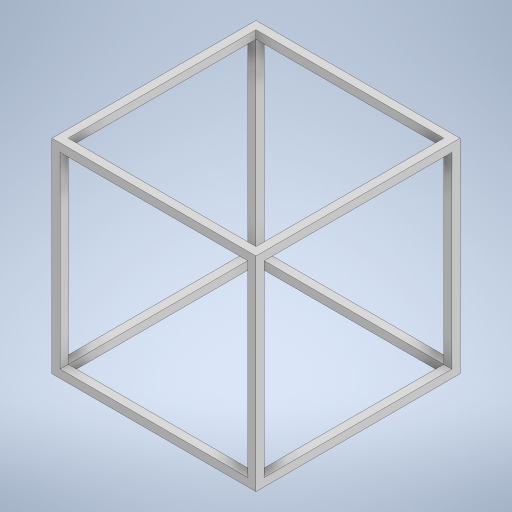
# Autodesk Inventor part: wymiar
Saved by Autodesk Inventor 2023.5 (Build 275446000, 446)
## iProperties
Created: 2025-03-17
Part Number: wymiar
Material: Ogólny
Document SubType Name: Modeling
Designer: kamil
Density: 1 g/cm^3
Appearance: Domyślna
Author: kamil
Autodesk Inventor part; units mm, degrees
ref_plane "YZ Plane" through (0, 0, 0) normal (1, 0, 0) x (0, 1, 0)
ref_plane "XZ Plane" through (0, 0, 0) normal (0, 1, 0) x (-1, 0, 0)
ref_plane "XY Plane" through (0, 0, 0) normal (0, 0, 1) x (1, 0, 0)
sketch "Szkic1" plane through (0, 0, 0) normal (0, 1, 0) x (-1, 0, 0)
  line L0 (0, 0) -> (-50, 0)
  line L1 (-50, 0) -> (-50, -50)
  line L2 (-50, -50) -> (0, -50)
  line L3 (0, -50) -> (0, 0)
  line L4 (-2, -2) -> (-48, -2)
  line L5 (-48, -2) -> (-48, -48)
  line L6 (-48, -48) -> (-2, -48)
  line L7 (-2, -48) -> (-2, -2)
  dimension "d0" = 50
  dimension "d1" = 50
  dimension "d2" = 2
  constraints: 16 end point, 4 parallel, 2 perpendicular, 1 horizontal, 3 other
  measures "d0" distance of L2.end L1.end
  measures "d1" distance of L2.end L0.start
  measures "d2" distance between parallel lines of L3 L7
extrude "Wyciągnięcie proste1" add sketch "Szkic1" along normal blind 2
sketch "Szkic2" plane through (0, 2, 0) normal (0, 1, 0) x (1, 0, 0)
  line L0 (50, 0) -> (50, 50) projected
  line L1 (50, 50) -> (0, 50) projected
  line L2 (0, 50) -> (0, 0) projected
  line L3 (0, 0) -> (50, 0) projected
  line L4 (2, 2) -> (2, 48) projected
  line L5 (2, 48) -> (48, 48) projected
  line L6 (48, 48) -> (48, 2) projected
  line L7 (48, 2) -> (2, 2) projected
  line L8 (0, 50) -> (0, 0) projected
  line L9 (0, 0) -> (2, 0)
  line L10 (2, 0) -> (2, 2)
  line L11 (2, 2) -> (0, 2)
  line L12 (0, 2) -> (0, 0)
  line L13 (2, 48) -> (0, 48)
  line L14 (0, 48) -> (0, 50)
  line L15 (0, 50) -> (2, 50)
  line L16 (2, 50) -> (2, 48)
  line L17 (0, 0) -> (50, 0) projected
  line L18 (50, 0) -> (48, 0)
  line L19 (48, 0) -> (48, 2)
  line L20 (48, 2) -> (50, 2)
  line L21 (50, 2) -> (50, 0)
  line L22 (2, 48) -> (48, 48) projected
  line L23 (48, 48) -> (50, 48)
  line L24 (50, 48) -> (50, 50)
  line L25 (50, 50) -> (48, 50)
  line L26 (48, 50) -> (48, 48)
  constraints: 32 end point, 8 parallel, 4 horizontal, 4 perpendicular
extrude "Wyciągnięcie proste2" add sketch "Szkic2" along normal blind 46 contours L3 L19 L20 L0 | L23 L26 L1 L0 | L3 L2 L11 L10 | L13 L2 L1 L16
sketch "Szkic3" plane through (0, 48, 0) normal (0, 1, 0) x (1, 0, 0)
  line L0 (48, 50) -> (2, 50) projected
  line L1 (50, 0) -> (50, 50) projected
  line L2 (0, 0) -> (50, 0) projected
  line L3 (0, 50) -> (0, 0) projected
  line L4 (50, 50) -> (0, 50) projected
  line L5 (2, 2) -> (2, 48) projected
  line L6 (48, 2) -> (2, 2) projected
  line L7 (48, 48) -> (48, 2) projected
  line L8 (2, 48) -> (48, 48) projected
extrude "Wyciągnięcie proste3" add sketch "Szkic3" along normal blind 2
